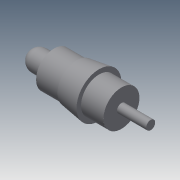
# Autodesk Inventor part: VN-3-1
Saved by Autodesk Inventor 2015 SP1 (Build 190203100, 203)
## iProperties
Created: 2015-05-25
Part Number: VN-3-1
Material: Generic
Document SubType Name: Modeling
Designer: Yamaura
Density: 1 g/cm^3
Appearance: Default
Author: Yamaura
Autodesk Inventor part; units mm, degrees
ref_plane "YZ Plane" through (0, 0, 0) normal (1, 0, 0) x (0, 1, 0)
ref_plane "XZ Plane" through (0, 0, 0) normal (0, 1, 0) x (-1, 0, 0)
ref_plane "XY Plane" through (0, 0, 0) normal (0, 0, 1) x (1, 0, 0)
sketch "スケッチ1" plane through (0, 0, 0) normal (0, 0, 1) x (1, 0, 0)
  line L0 (0, 0) -> (-4.1, 0)
  line L1 (-4.1, 0) -> (-4.1, 0.45)
  line L2 (-4.1, 0.45) -> (0, 0.45)
  line L3 (0, 0.45) -> (0, 0)
  dimension "d0" = 4.1
  dimension "d1" = 0.45
  constraints: 8 end point, 2 parallel, 1 horizontal, 1 perpendicular
  measures "d0" distance of L1.end L2.end
  measures "d1" distance of L0.end L1.end
revolve "回転1" add sketch "スケッチ1" angle 360 about axis through (0, 0, 0) along (-1, 0, 0)
sketch "スケッチ2" plane through (0, 0, 0) normal (0, 0, 1) x (1, 0, 0)
  line L0 (0, 0) -> (1.3, 0)
  line L1 (1.3, 0) -> (1.3, 0.2)
  line L2 (1.3, 0.2) -> (0, 0.2)
  line L3 (0, 0.2) -> (0, 0)
  dimension "d3" = 1.3
  dimension "d4" = 0.2
  constraints: 8 end point, 2 parallel, 1 horizontal, 1 perpendicular
  measures "d3" distance of L2.end L1.end
  measures "d4" distance of L1.end L0.end
revolve "回転2" add sketch "スケッチ2" angle 360 about axis through (0, 0, 0) along (1, 0, 0)
sketch "スケッチ3" plane through (0, 0, 0) normal (0, 0, 1) x (1, 0, 0)
  line L0 (0, 0) -> (-3, 0)
  line L1 (-3, 0) -> (-3, 0.8)
  line L2 (-3, 0.8) -> (0, 0.8)
  line L3 (0, 0.8) -> (0, 0)
  dimension "d6" = 3
  dimension "d7" = 0.8
  constraints: 8 end point, 2 parallel, 1 horizontal, 1 perpendicular
  measures "d6" distance of L1.end L2.end
  measures "d7" distance of L0.end L1.end
revolve "回転3" add sketch "スケッチ3" angle 360 about axis through (0, 0, 0) along (-1, 0, 0)
sketch "スケッチ4" plane through (0, 0, 0) normal (0, 0, 1) x (1, 0, 0)
  line L0 (-2, 0) -> (-2, 0.85)
  line L1 (-2, 0.85) -> (-1, 1)
  line L2 (-1, 1) -> (-1, 0)
  line L3 (-1, 0) -> (-2, 0)
  line L4 (0, -5.0705) -> (0, 2.4355) projected
  line L5 (-5.18, 0) -> (2.38, 0) projected
  point P0 (0, 0)
  dimension "d9" = 2
  dimension "d10" = 1
  dimension "d11" = 0.85
  dimension "d12" = 1
  constraints: 8 end point, 1 collinear, 1 parallel, 1 perpendicular, 1 vertical
  measures "d9" distance from line of L0 point (0, 0)
  measures "d10" distance between parallel lines of L2 L0
  measures "d11" distance of L0.start L0.end
  measures "d12" distance of L1.end L2.end
revolve "回転4" add sketch "スケッチ4" angle 360 about axis through (-1, 0, 0) along (-1, 0, 0)
fillet "フィレット1" radius 0.45 1 edges at (-4.1, -0.45, 0)
